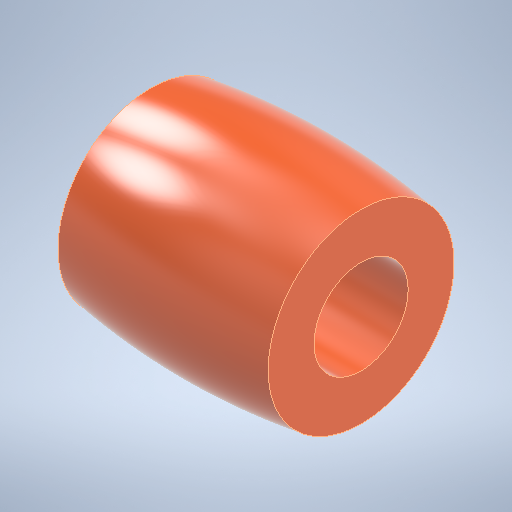
# Autodesk Inventor part: 3D_taru-core
Saved by Autodesk Inventor 2025 (Build 290162000, 162)
## iProperties
Created: 2024-06-25
Part Number: 3D_taru-core
Material: 一般
Document SubType Name: Modeling
Designer: 8326d
Density: 1 g/cm^3
Appearance: 滑らか - 淡いオレンジ
Author: 8326d
## iProperties of the stored document 3D_taru-core_3D プリント.ipt
Created: 2024-07-27
Part Number: 3D_taru-core_3D プリント
Material: 一般
Document SubType Name: Modeling
Designer: 8326d
Density: 1 g/cm^3
Appearance: 既定
Author: 8326d
Autodesk Inventor part; units mm, degrees
ref_plane "YZ Plane" through (0, 0, 0) normal (1, 0, 0) x (0, 1, 0)
ref_plane "XZ Plane" through (0, 0, 0) normal (0, 1, 0) x (-1, 0, 0)
ref_plane "XY Plane" through (0, 0, 0) normal (0, 0, 1) x (1, 0, 0)
sketch "スケッチ1" plane through (0, 0, 0) normal (0, 0, 1) x (1, 0, 0)
  line L0 (-6.2586, 26.5) -> (6.2586, 26.5)
  line L1 (6.2586, 26.5) -> (6.2586, 36.5)
  line L2 (6.2586, 36.5) -> (-6.2586, 36.5)
  line L3 (-6.2586, 36.5) -> (-6.2586, 26.5)
  line L4 (-6.2586, 26.5) -> (6.2586, 36.5) construction
  line L5 (6.2586, 26.5) -> (-6.2586, 36.5) construction
  line L6 (-6.2586, 36.5) -> (0, 0) construction
  line L7 (0, 0) -> (0, 36.5) construction
  circle A0 centre (0, 0) radius 35 construction
  line L8 (-5.6586, 36.5) -> (-5.6586, 26.5)
  arc A1 (5.6586, 36.5) -> (-5.6586, 36.5) centre (0, 0) ccw
  line L9 (5.6586, 26.5) -> (5.6586, 36.5)
  line L10 (-5.6586, 31.5) -> (5.6586, 31.5)
  line L11 (-5.6586, 34.03) -> (5.6586, 34.03)
  point P0 (0, 31.5)
  dimension "d0" = 31.5
  dimension "d1" = 9.73
  dimension "d2" = 70
  dimension "d3" = 1.5
  dimension "d4" = 0.6
  dimension "d6" = 0.6
  dimension "d7" = 2.53
  constraints: 24 end point, 7 point on line, 5 midpoint, 4 perpendicular, 3 coincident, 2 centre point, 2 parallel, 2 point on circle, 1 horizontal, 1 vertical alignment
  measures "d0" distance of point (0, 0) point (0, 31.5)
  measures "d1" angle of L6 L7
  measures "d2" diameter of A0
  measures "d3" distance edge to line of A0 L2
  measures "d4" distance between parallel lines of L3 L8
  measures "d6" distance between parallel lines of L1 L9
  measures "d7" distance between parallel lines of L10 L11
revolve "回転1" add sketch "スケッチ1" angle 360 about axis through (-5.6586, 31.5, 0) along (1, 0, 0) contours A1 L2 | L2 L9 L11 L8
equation "\"d0\" = 0.9 * r"
equation "\"d2\" = 2 * r"
equation "\"d6\" = d4"
equation "\"r\" = 35"
